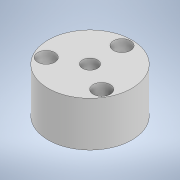
# Autodesk Inventor part: table
Saved by Autodesk Inventor 2020 (Build 240168000, 168)
## iProperties
Created: 2019-06-14
Part Number: table
Material: Generic
Document SubType Name: Modeling
Designer: ColinP
Density: 1 g/cm^3
Appearance: Default
Mass: 11.1656 g
Surface Area: 41.7742 cm^2
Volume: 11.1656 cm^3
Author: ColinP
Autodesk Inventor part; units mm, degrees
ref_plane "YZ Plane" through (0, 0, 0) normal (1, 0, 0) x (0, 1, 0)
ref_plane "XZ Plane" through (0, 0, 0) normal (0, 1, 0) x (-1, 0, 0)
ref_plane "XY Plane" through (0, 0, 0) normal (0, 0, 1) x (1, 0, 0)
sketch "Sketch1" plane through (0, 0, 0) normal (0, 1, 0) x (-1, 0, 0)
  line L0 (0, 0) -> (13.6144, 0)
  circle A0 centre (0, 0) radius 17.78
  dimension "d0" = 13.6144
  dimension "d1" = 35.56
  constraints: 2 coincident, 2 end point, 1 centre point, 1 horizontal
  measures "d0" distance of L0.start L0.end
  measures "d1" diameter of A0
extrude "Extrusion1" add sketch "Sketch1" along normal blind 19.05
sketch "Sketch3" plane through (0, 19.05, 0) normal (0, 1, 0) x (1, 0, 0)
  line L0 (0, 0) -> (0, 13.6144)
  line L1 (0, 0) -> (13.6144, 0) construction
  dimension "d4" = 13.6144
  dimension "d5" = 90
  constraints: 4 end point, 1 horizontal, 1 perpendicular, 1 vertical
  measures "d4" distance of L0.start L0.end
  measures "d5" angle of L1 L0
hole "Hole1" at (0, 19.05, -13.6144) direction (0, -1, 0) diameter 4.9022 end through all counterbore diameter 7.239 counterbore depth 5.08
sketch "Sketch4" plane through (0, 0, 0) normal (0, -1, 0) x (1, 0, 0)
  circle A0 centre (0, -13.6144) radius 2.4511 projected
  line L0 (0, 0) -> (0, -13.6144)
  constraints: 2 end point, 1 vertical
hole "Hole2" at (0, 0, -13.6144) direction (0, 1, 0) diameter 4.9022 depth 6.35 counterbore diameter 6.5532 counterbore depth 1.6002
pattern_circular "Circular Pattern1" count 3 over 360 about axis through (0, 0, 0) along (0, 1, 0) of "Hole1", "Hole2"
sketch "Sketch6" plane through (0, 19.05, 0) normal (0, 1, 0) x (1, 0, 0)
  point P0 (0, 0)
  point P1 (0, 0)
  constraints: 1 coincident
hole "Hole3" at (0, 19.05, 0) direction (0, -1, 0) diameter 6.35 end through all
body "Solid1"
